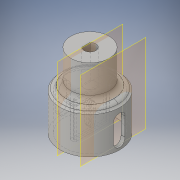
# Autodesk Inventor part: Autofeeder part 1
Saved by Autodesk Inventor 2016 (Build 200138000, 138)
## iProperties
Created: 2016-12-02
Part Number: Autofeeder part 1
Material: Generic
Document SubType Name: Modeling
Designer: Student
Density: 1 g/cm^3
Appearance: Default
Author: Student
Autodesk Inventor part; units mm, degrees
ref_plane "XZ Plane" through (0, 0, 0) normal (0, 1, 0) x (-1, 0, 0)
ref_plane "XY Plane" through (0, 0, 0) normal (0, 0, 1) x (1, 0, 0)
sketch "Sketch1" plane through (0, 0, 0) normal (0, 1, 0) x (-1, 0, 0)
  circle A0 centre (0, 0) radius 3.2318
  line L0 (2.28, 2.2905) -> (2.28, -2.2905)
  circle A1 centre (0, 0) radius 10.5918
  dimension "d2" = 5.5118
  dimension "d3" = 21.1836
  constraints: 2 centre point, 2 coincident, 2 end point, 2 point on circle, 1 vertical
  measures "d3" diameter of A1
extrude "Extrusion1" add sketch "Sketch1" along normal blind 18.034 contours A0 L0 | A1 picked at (2.4147, -0.6)
sketch "Sketch2" plane through (0, 0, 0) normal (0, -1, 0) x (1, 0, 0)
  circle A0 centre (0, 0) radius 15.24
  dimension "d6" = 30.48
  constraints: 1 centre point, 1 coincident
  measures "d6" diameter of A0
extrude "Extrusion2" add sketch "Sketch2" along normal blind 2.54
sketch "Sketch3" plane through (0, -2.54, 0) normal (0, -1, 0) x (1, 0, 0)
  circle A0 centre (0, 0) radius 14.351
  circle A1 centre (0, 0) radius 16.4291
  dimension "d9" = 28.702
  constraints: 2 centre point, 2 coincident
  measures "d9" diameter of A0
extrude "Extrusion3" add sketch "Sketch3" along normal blind 20.32
sketch "Sketch4" plane through (0, -2.54, 0) normal (0, -1, 0) x (1, 0, 0)
  line L0 (-0.4572, -8.89) -> (0.4572, -8.89)
  line L1 (0.4572, -8.89) -> (0.4572, 8.89)
  line L2 (0.4572, 8.89) -> (-0.4572, 8.89)
  line L3 (-0.4572, 8.89) -> (-0.4572, -8.89)
  line L4 (-0.4572, -8.89) -> (0.4572, 8.89) construction
  line L5 (0.4572, -8.89) -> (-0.4572, 8.89) construction
  line L6 (-1.524, -9.9568) -> (1.524, -9.9568)
  line L7 (1.524, -9.9568) -> (1.524, 9.9568)
  line L8 (1.524, 9.9568) -> (-1.524, 9.9568)
  line L9 (-1.524, 9.9568) -> (-1.524, -9.9568)
  point P0 (0, 0)
  dimension "d24" = 0.9144
  dimension "d25" = 17.78
  dimension "d26" = 1.0668
  constraints: 20 end point, 4 parallel, 2 midpoint, 2 perpendicular, 1 horizontal, 3 other
  measures "d24" distance of L2.end L1.end
  measures "d25" distance of L1.end L0.end
  measures "d26" distance between parallel lines of L3 L9
extrude "Extrusion4" add sketch "Sketch4" along normal blind 19.177
fillet "Fillet3" radius 2.54 1 edges at (10.5918, 0, 0)
fillet "Fillet4" radius 2.54 1 edges at (-15.24, -2.54, 0)
fillet "Fillet5" radius 2.54 1 edges at (-15.24, 0, 0)
fillet "Fillet7" radius 0.762 4 edges at (1.524, -12.1285, 9.9568) (-1.524, -12.1285, 9.9568) (-1.524, -12.1285, -9.9568) (1.524, -12.1285, -9.9568)
fillet "Fillet8" radius 2.54 8 edges at (1.3008, -2.54, -9.7336) (0, -2.54, -9.9568) (-1.3008, -2.54, -9.7336) (-1.524, -2.54, 0) (-1.3008, -2.54, 9.7336) (0, -2.54, 9.9568) (1.3008, -2.54, 9.7336) (1.524, -2.54, 0)
sketch "Sketch5" plane through (0, 0, 0) normal (1, 0, 0) x (0, 1, 0)
  line L0 (-18.4785, 0) -> (-8.3185, 0) construction
  line L1 (-18.4785, -1.27) -> (-8.3185, -1.27)
  line L2 (-8.3185, 1.27) -> (-18.4785, 1.27)
  arc A0 (-18.4785, 1.27) -> (-18.4785, -1.27) centre (-18.4785, 0) ccw
  arc A1 (-8.3185, -1.27) -> (-8.3185, 1.27) centre (-8.3185, 0) ccw
  line L3 (-21.717, -9.9568) -> (-5.08, -9.9568) projected
  line L4 (0, -3.2318) -> (0, 3.2318) projected
  point P0 (0, 0)
  point P1 (-13.3985, 0)
  point P2 (-13.3985, -9.9568)
  point P3 (0, 0)
  point P4 (0, 2.2905)
  point P5 (0, -2.2905)
  dimension "d29" = 2.54
  dimension "d30" = 12.7
  constraints: 8 end point, 4 point on circle, 4 tangent, 3 midpoint, 2 centre point, 1 horizontal, 1 horizontal alignment, 1 parallel, 1 vertical alignment
  measures "d29" diameter of A1
extrude "Extrusion5" cut sketch "Sketch5" along normal mid plane 25.4
ref_plane "Work Plane1" through (12.7, 0, 0) normal (1, 0, 0) x (0, 1, 0)
sketch "Sketch6" plane through (12.7, 0, 0) normal (1, 0, 0) x (0, 1, 0)
  arc A0 (-8.3185, -1.27) -> (-8.3185, 1.27) centre (-8.3185, 0) ccw construction
  arc A1 (-18.4785, 1.27) -> (-18.4785, -1.27) centre (-18.4785, 0) ccw construction
  line L0 (-18.4785, 1.27) -> (-8.3185, 1.27) construction
  line L1 (-8.3185, -1.27) -> (-18.4785, -1.27) construction
  arc A2 (-8.3185, -3.175) -> (-8.3185, 3.175) centre (-8.3185, 0) ccw
  line L2 (-8.3185, -3.175) -> (-18.4785, -3.175)
  arc A3 (-18.4785, 3.175) -> (-18.4785, -3.175) centre (-18.4785, 0) ccw
  line L3 (-18.4785, 3.175) -> (-8.3185, 3.175)
  point P0 (0, 0)
  dimension "d34" = 3.175
  constraints: 8 end point, 8 point on circle, 4 centre point, 3 other
  measures "d34" distance from line of A1.centre L3
extrude "Extrusion6" cut sketch "Sketch6" along normal blind 25.4
mirror "Mirror1" about plane through (0, 0, 0) normal (1, 0, 0) of "Extrusion6"
body "Solid1"
